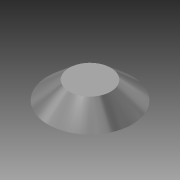
# Autodesk Inventor part: 3628_
Saved by Autodesk Inventor 2013 (Build 170138000, 138)
## iProperties
Category: PARTsolutions
Company: 8020
Created: 2013-09-15
Part Number: 3628_
Catalog Web Link: www.cadenas.de
Description: 3265, 3268-Countersunk Bolt
Vendor: 8020
Document SubType Name: Modeling
Designer: PARTuser1
Manufacturer: 8020
Density: 8.08 g/cm^3
Material: Stainless Steel
Mass: 0.656797 g
Surface Area: 1.86203 cm^2
Volume: 0.0812868 cm^3
PSOL_IDENT_0: {$CADENAS_DATA\23d-libs\8020\inch\linear_motion\csunk_bolt.prj},147 {VTYP=3D},{NB=3628_},{LINA=3628_
PSOL_IDENT_1: },{NN=3265, 3268},{DATE=22.08.2012},{GEOMDATE=15.06.2012 12:48:30},{VERSION=},{LINEID=50},{LINESUBID
PSOL_IDENT_2: =-1},{WBVAR=}  {NB=3628_},{LINA=3628_},{KT=DUMMY},{PN=3628},{PN1=10-24},{A=1.500},{TH=0.250},{CS=0.3
PSOL_IDENT_3: 85},{HD1=0.201}
CNS_NT: Countersunk Bolt
CNS_NB: 3628_
CNS_NBSYN: $PN._
CNS_LINA: 3628_
CNS_PN: 3628
CNS_PN1: 10-24
CNS_A: 1.500
CNS_TH: 0.250
CNS_CS: 0.385
CNS_HD1: 0.201
SUPPLIER: 8020
ARTICLENO: 3628_
BOMINFO: 3628_
CREATOR: CADENAS GmbH
Title: 3628_
Author: Cadenas PARTsolutions
Comments: Countersunk Bolt
Autodesk Inventor part; units mm, degrees
sketch "Sketch_3" plane through (0, 0, 0) normal (0, 0, 1) x (1, 0, 0)
  line L0 (0, -1.9608) -> (0, 0.1172)
  line L1 (0, 0.1172) -> (2.413, 0.1172)
  line L2 (2.413, 0.1172) -> (4.8895, -1.9608)
  line L3 (4.8895, -1.9608) -> (0, -1.9608)
  line L4 (0, -1.9608) -> (0, 0.1172)
  constraints: 10 end point
revolve "Revolution1" add sketch "Sketch_3" angle 360 about axis through (0, -1.9608, 0) along (0, -1, 0)
sketch "Sketch_4" plane through (0, -1.9608, 0) normal (0, -1, 0) x (1, 0, 0)
  line L0 (-2.5883, -0.5283) -> (-0.7823, -0.5283)
  arc A0 (-0.5283, -0.7823) -> (-0.7823, -0.5283) centre (-0.7823, -0.7823) ccw
  line L1 (-0.5283, -0.7823) -> (-0.5283, -2.5883)
  line L2 (-0.5283, -2.5883) -> (0.5283, -2.5883)
  line L3 (0.5283, -2.5883) -> (0.5283, -0.7823)
  arc A1 (0.7823, -0.5283) -> (0.5283, -0.7823) centre (0.7823, -0.7823) ccw
  line L4 (0.7823, -0.5283) -> (2.5883, -0.5283)
  line L5 (2.5883, -0.5283) -> (2.5883, 0.5283)
  line L6 (2.5883, 0.5283) -> (0.7823, 0.5283)
  arc A2 (0.5283, 0.7823) -> (0.7823, 0.5283) centre (0.7823, 0.7823) ccw
  line L7 (0.5283, 0.7823) -> (0.5283, 2.5883)
  line L8 (0.5283, 2.5883) -> (-0.5283, 2.5883)
  line L9 (-0.5283, 2.5883) -> (-0.5283, 0.7823)
  arc A3 (-0.7823, 0.5283) -> (-0.5283, 0.7823) centre (-0.7823, 0.7823) ccw
  line L10 (-0.7823, 0.5283) -> (-2.5883, 0.5283)
  line L11 (-2.5883, 0.5283) -> (-2.5883, -0.5283)
  constraints: 24 end point, 8 point on circle, 4 centre point
extrude "Extrusion1" cut sketch "Sketch_4" against normal blind 0.9195
ref_plane "screw_XY" through (0, 0, 0) normal (0, 1, 0) x (1, 0, 0)
ref_plane "screw_YZ" through (0, 0, 0) normal (1, 0, 0) x (0, 0, -1)
ref_plane "screw_ZX" through (0, 0, 0) normal (0, 0, -1) x (0, 1, 0)
body "Solid1"
